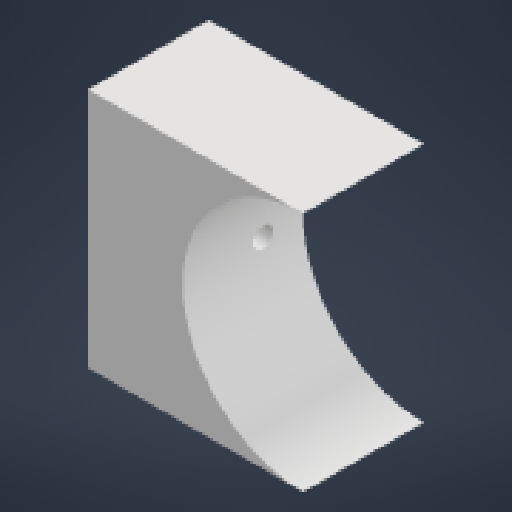
# Autodesk Inventor part: Part27
Saved by Autodesk Inventor 2027.1 (Build 311270010, 270A)
## iProperties
Created: 2026-10-02
Part Number: Part27
Material: Generic
Document SubType Name: Modeling
Designer: daniel
Density: 1 g/cm^3
Appearance: Default
Author: daniel
Autodesk Inventor part; units mm, degrees
ref_plane "YZ Plane" through (0, 0, 0) normal (1, 0, 0) x (0, 1, 0)
ref_plane "XZ Plane" through (0, 0, 0) normal (0, 1, 0) x (-1, 0, 0)
ref_plane "XY Plane" through (0, 0, 0) normal (0, 0, 1) x (1, 0, 0)
sketch "Sketch1" plane through (0, 0, 0) normal (0, 0, 1) x (1, 0, 0)
  line L0 (7.8735, 17.8984) -> (31.3735, 17.8984)
  line L1 (31.3735, 17.8984) -> (31.3735, -42.1016)
  line L2 (31.3735, -42.1016) -> (7.8735, -42.1016)
  line L3 (7.8735, -42.1016) -> (7.8735, 17.8984)
  circle A0 centre (61.3735, -12.1016) radius 30
  line L4 (61.3735, 17.8984) -> (31.3735, 17.8984)
  line L5 (61.3735, -42.1016) -> (31.3735, -42.1016)
  point P0 (0, 0)
  point P1 (7.8735, -12.1016)
  dimension "d1" = 60
  dimension "d2" = 60
  dimension "d3" = 53.5
  constraints: 12 end point, 2 horizontal, 2 parallel, 2 point on circle, 2 tangent, 1 centre point, 1 midpoint, 1 perpendicular
  measures "d1" distance of L0.end L1.end
  measures "d2" diameter of A0
  measures "d3" distance of point (7.874, -12.102) A0.centre
extrude "Extrusion1" add sketch "Sketch1" along normal blind 30 contours L0 L1 L2 L3 | L4 A0 L1 | A0 L5 L1
sketch "Sketch2" plane through (7.8735, -42.1016, 0) normal (-1, 0, 0) x (0, 0, 1)
  circle A0 centre (10, 30) radius 2.5
  line L0 (0, 60) -> (0, 0) projected
  line L1 (0, 0) -> (30, 0) projected
  point P0 (0, 42.1016)
  point P1 (0, 30)
  dimension "d6" = 5
  dimension "d7" = 10
  dimension "d8" = 30
  constraints: 1 centre point, 1 midpoint
  measures "d6" diameter of A0
  measures "d7" distance of point (0, 30) A0.centre
  measures "d8" distance from line of L1 A0.centre
extrude "Extrusion2" cut sketch "Sketch2" against normal blind 30
body "Solid1"
